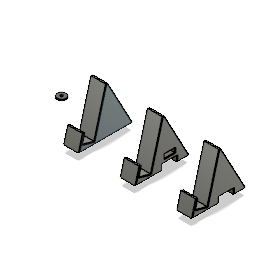
CD Jew Case Display Stand v5 (Autodesk Fusion 360 design; units mm, degrees)
Autodesk Fusion 360 part; units mm, degrees
sketch "Sketch1" plane through (0, 0, 0) normal (1, 0, 0) x (0, 0, -1)
  line L0 (0, 0) -> (-10.6, 0)
  line L1 (-10.6, 0) -> (-10.6, -2)
  line L2 (-10.6, -2) -> (0, -2)
  line L3 (0, -2) -> (0, 0)
  line L4 (-10.6, -2) -> (-12.6, -2)
  line L5 (-12.6, -2) -> (-12.6, 8)
  line L6 (-12.6, 8) -> (-10.6, 8)
  line L7 (-10.6, 8) -> (-10.6, -2)
  line L8 (0, -2) -> (2, -2)
  line L9 (2, -2) -> (2, 40)
  line L10 (2, 40) -> (0, 40)
  line L11 (0, 40) -> (0, -2)
  dimension "d1" = 10.6
  dimension "d2" = 2
  dimension "d3" = 2
  dimension "d4" = 10
  dimension "d5" = 2
  dimension "d6" = 42
  constraint horizontal L0
  constraint vertical L1
  constraint horizontal L2
  constraint vertical L3
  constraint coincident L0.start L3.end
  constraint horizontal L4
  constraint vertical L5
  constraint horizontal L6
  constraint vertical L7
  constraint horizontal L8
  constraint vertical L9
  constraint horizontal L10
  constraint vertical L11
  measures "d1" distance of L0.start L0.end
  measures "d2" distance of L0.start L2.end
  measures "d3" distance of L1.end L4.end
  measures "d4" distance of L1.end L6.end
  measures "d5" distance of L2.end L8.end
  measures "d6" distance of L2.end L10.end
extrude "Extrude1" add sketch "Sketch1" along normal blind 2 makes body 1
move_body "Move1" bodies 1 to x (1, 0, 0) y (0, 0.965926, -0.258819) z (0, 0.258819, 0.965926) at (0, 0.4495, -0.5858)
sketch "Sketch2" plane through (2, 0, 0) normal (1, 0, 0) x (0, 0, -1)
  line L0 (-12.1025, 1.7788) -> (2, -2)
  line L1 (2, -2) -> (12.8704, 38.5689)
  line L2 (12.8704, 38.5689) -> (10.9385, 39.0865)
  line L3 (10.9385, 39.0865) -> (0.5858, 0.4495)
  line L4 (0.5858, 0.4495) -> (-9.653, 3.193)
  line L5 (-9.653, 3.193) -> (-7.5825, 10.9204)
  line L6 (-7.5825, 10.9204) -> (-9.5143, 11.438)
  line L7 (-9.5143, 11.438) -> (-12.1025, 1.7788)
  line L8 (2, -2) -> (-13.115, -2)
  line L9 (-13.115, -2) -> (-12.1025, 1.7788)
  line L10 (2, -2) -> (32, -2)
  arc A0 (12.8704, 38.5689) -> (32, -2) centre (69.4566, 40.4566) ccw
  line L11 (12.8704, 38.5689) -> (32, -2)
  dimension "d9" = 30
  constraint coincident L0.end L1.start
  constraint horizontal L8
  constraint coincident L0.start L7.end
  constraint perpendicular L0 L9
  constraint horizontal L10
  constraint coincident L1.end L2.start
  measures "d9" distance of L0.end L10.end
extrude "Extrude2" add sketch "Sketch2" against normal blind 2 contours L0 L8 L9 | L1 L10 A0 | A0 L11 bodies 1
draft "Draft1" angle 3 neutral plane through (0, 38.5689, -12.8704) pull (0, 0.965926, -0.258819) 1 faces at (1.3333, 25.0459, -19.2469) on bodies 1
sketch "Sketch3" plane through (2, 0, 0) normal (1, 0, 0) x (0, 0, -1)
  line L0 (12.8704, 38.5689) -> (10.9385, 39.0865)
  line L1 (10.9385, 39.0865) -> (0.5858, 0.4495)
  line L2 (0.5858, 0.4495) -> (-9.653, 3.193)
  line L3 (-9.653, 3.193) -> (-7.5825, 10.9204)
  line L4 (-7.5825, 10.9204) -> (-9.5143, 11.438)
  line L5 (-9.5143, 11.438) -> (-13.115, -2)
  line L6 (-13.115, -2) -> (34.6647, -2)
  line L7 (34.6647, -2) -> (34.6647, 3)
  line L8 (34.6647, 3) -> (34.6647, 4)
  line L9 (34.6647, 4) -> (34.6647, 7.25)
  line L10 (34.6647, 7.25) -> (34.6647, 10.75)
  line L11 (34.6647, 10.75) -> (23.923, 10.75)
  line L12 (23.923, 10.75) -> (21.923, 10.75)
  line L13 (21.923, 10.75) -> (12.723, 10.75)
  line L14 (12.723, 10.75) -> (12.723, 7.25)
  line L15 (12.723, 7.25) -> (21.923, 7.25)
  line L16 (21.923, 7.25) -> (21.923, 10.75)
  line L17 (17.323, 7.25) -> (17.323, 4)
  line L18 (17.323, 4) -> (23.823, 4)
  line L19 (23.823, 4) -> (10.823, 4)
  line L20 (10.823, 4) -> (10.823, -2)
  line L21 (10.823, -2) -> (23.823, -2)
  line L22 (23.823, -2) -> (23.823, 4)
  line L23 (34.6647, -2) -> (12.8704, 38.5689)
  dimension "d12" = 5
  dimension "d13" = 3.25
  dimension "d14" = 3.5
  dimension "d15" = 2
  dimension "d16" = 9.2
  dimension "d17" = 3.5
  dimension "d18" = 3.25
  dimension "d19" = 6.5
  dimension "d20" = 13
  constraint coincident L6.end L7.start
  constraint perpendicular L6 L7
  constraint parallel L7 L8
  constraint parallel L8 L9
  constraint parallel L9 L10
  constraint perpendicular L10 L11
  constraint perpendicular L10 L12
  constraint horizontal L13
  constraint vertical L14
  constraint horizontal L15
  constraint vertical L16
  constraint midpoint L15 L17.start
  constraint perpendicular L15 L17
  constraint perpendicular L17 L18
  constraint horizontal L19
  constraint vertical L20
  constraint horizontal L21
  constraint vertical L22
  measures "d12" distance of L6.end L7.end
  measures "d13" distance of L8.end L9.end
  measures "d14" distance of L9.end L10.end
  measures "d15" distance of L11.end L12.end
  measures "d16" distance of L12.end L13.end
  measures "d17" distance of L12.end L15.end
  measures "d18" distance of L17.start L17.end
  measures "d19" distance of L17.end L18.end
  measures "d20" distance of L18.end L19.end
extrude "Extrude3" add 1 faces at (0, 12.3395, -16.0403) along direction (-1, 0, 0) blind 12 on bodies 1 bodies 1
copy_body "CopyPasteBodies1" bodies 1 makes body 2
move_body "Move2" bodies 2 to x (1, 0, 0) y (0, 1, 0) z (0, 0, 1) at (-50, 0, 0)
copy_body "CopyPasteBodies2" bodies 1 2 makes body 3 makes body 4
move_body "Move3" bodies 3 4 to x (1, 0, 0) y (0, 1, 0) z (0, 0, 1) at (-100, 0, 0)
extrude "Extrude4" cut sketch "Sketch3" against normal blind 64 contours L13 L14 L15 L16 | L6 L18 L19 L20 L21 L22 bodies 1 2
extrude "Extrude5" add sketch "Sketch3" against normal blind 2 contours L13 L14 L15 L16 bodies 1
extrude "Extrude6" add sketch "Sketch3" along normal blind -64 and the other way blind 62 contours L13 L14 L15 L16 bodies 2
sketch "Sketch4" plane through (0, 0, 0) normal (0, 1, 0) x (1, 0, 0)
  circle A0 centre (28.667, 5.442) radius 10.4527
  ellipse E0 centre (28.667, 5.442) end of major axis (31.6436, 5.442) minor radius 2.9766
  point P0 (39.1197, 5.442)
  point P1 (31.6436, 5.442)
extrude "Extrude7" add sketch "Sketch4" along normal blind 3 separate body makes body 5
scale "Scale1" factor 0.382665 about (39.1197, 0, -5.442) bodies 5
move_body "Move4" bodies 5 to x (1, 0, 0) y (0, 1, 0) z (0, 0, 1) at (-33.1198, -2, -23.8018)
move_body "Move5" bodies 5 to x (1, 0, 0) y (0, 1, 0) z (0, 0, 1) at (-7, -5, 0)
extrude "Extrude8" cut 1 faces at (-5, -5.852, -32.2827) along direction (0, 1, 0) blind 4.352 on bodies 5 bodies 1
extrude "Extrude9" cut 1 faces at (-5.3459, -2, -29.0223) along direction (0, 1, 0) blind 1 on bodies 1 bodies 1
move_body "Move6" bodies 5 to x (1, 0, 0) y (0, 1, 0) z (0, 0, 1) at (-43, 5, 0)
move_body "Move7" bodies 5 to x (1, 0, 0) y (0, 1, 0) z (0, 0, 1) at (-7, -5, 0)
extrude "Extrude10" cut 1 faces at (-55, -5.852, -32.2827) along direction (0, 1, 0) blind 4.352 on bodies 5 bodies 2
move_body "Move8" bodies 5 to x (1, 0, 0) y (0, 1, 0) z (0, 0, 1) at (-50, 5, -5.4209)
move_body "Move9" bodies 5 to x (1, 0, 0) y (0, 1, 0) z (0, 0, 1) at (0, -5, 6)
extrude "Extrude11" cut 1 faces at (-105, -5.852, -31.7035) along direction (0, 1, 0) blind 4.352 on bodies 5 bodies 3
move_body "Move10" bodies 5 to x (1, 0, 0) y (0, 1, 0) z (0, 0, 1) at (-50, 3.852, -6)
move_body "Move11" bodies 5 to x (1, 0, 0) y (0, 1, 0) z (0, 0, 1) at (0, -5, 6)
extrude "Extrude12" cut 1 faces at (-155, -7, -31.7035) along direction (0, 1, 0) blind 5.5 on bodies 5 bodies 4
extrude "Extrude13" cut 3 faces at (-155.3459, -2, -28.4431) (-105.3458, -2, -28.4429) (-55.3055, -2, -29.4529) along direction (0, 1, 0) blind 1 on bodies 2 3 4 bodies 2 3 4
delete_body "RemoveBody1" bodies 4
sketch "Sketch5" plane through (0, -2, 0) normal (0, -1, 0) x (1, 0, 0)
  line L0 (-62, -10.823) -> (-48, -10.823)
  line L1 (-48, -10.823) -> (-48, 13.115)
  line L2 (-48, 13.115) -> (-62, 13.115)
  line L3 (-62, 13.115) -> (-62, -10.823)
  line L4 (-62, 1.146) -> (-48, 1.146) construction
  line L5 (-48, 1.146) -> (-48, 13.115) construction
  line L6 (-48, 13.115) -> (-62, 13.115) construction
  line L7 (-62, 13.115) -> (-62, 1.146) construction
  text T0 "L" font "Arial" height 10 align centre middle in box 14 x 11.969 at (-62, 1.146) x (1, 0) y (0, 1) spacing 1 kerned
  constraint midpoint L1
  constraint coincident L2.end
sketch "Sketch6" plane through (0, -2, 0) normal (0, -1, 0) x (1, 0, 0)
  line L0 (-12, -10.823) -> (2, -10.823)
  line L1 (2, -10.823) -> (2, 13.115)
  line L2 (2, 13.115) -> (-12, 13.115)
  line L3 (-12, 13.115) -> (-12, -10.823)
  line L4 (-12, 1.146) -> (2, 1.146) construction
  line L5 (2, 1.146) -> (2, 13.115) construction
  line L6 (2, 13.115) -> (-12, 13.115) construction
  line L7 (-12, 13.115) -> (-12, 1.146) construction
  text T0 "R" font "Arial" height 10 align centre middle in box 14 x 11.969 at (-12, 1.146) x (1, 0) y (0, 1) spacing 1 kerned
  constraint midpoint L1
  constraint coincident L2.end
extrude "Extrude14" cut sketch "Sketch6" sketch "Sketch5" against normal blind 1 text T0 of sketch 2 text T0 bodies 1 2
sketch "Sketch7" plane through (0, 4, 0) normal (0, -1, 0) x (1, 0, 0)
  line L0 (-48, -23.823) -> (-48, -10.823)
  line L1 (-48, -10.823) -> (-62, -10.823)
  line L2 (-62, -10.823) -> (-62, -23.823)
  line L3 (-62, -23.823) -> (-48, -23.823)
  line L4 (-55, -10.823) -> (-55, -23.823)
  circle A0 centre (-55, -17.323) radius 2.4
  dimension "d50" = 4.8
  constraint midpoint L1 L4.start
  constraint midpoint L3 L4.end
  constraint midpoint L4 A0.centre
  measures "d50" diameter of A0
extrude "Extrude15" cut sketch "Sketch7" against normal blind 11 contours L4 A0 | L4 A0 bodies 2
sketch "Sketch8" plane through (0, 4, 0) normal (0, -1, 0) x (1, 0, 0)
  line L0 (-12, -10.823) -> (-12, -23.823)
  line L1 (-12, -23.823) -> (2, -23.823)
  line L2 (2, -23.823) -> (2, -10.823)
  line L3 (2, -10.823) -> (-12, -10.823)
  line L4 (-12, -17.323) -> (2, -17.323)
  circle A0 centre (-5, -17.323) radius 2.4
  dimension "d53" = 4.8
  constraint midpoint L0 L4.start
  constraint midpoint L2 L4.end
  constraint midpoint L4 A0.centre
  measures "d53" diameter of A0
extrude "Extrude16" cut sketch "Sketch8" against normal blind 11 contours L4 A0 | L4 A0 bodies 1
move_face "OffsetFaces1" offset -0.2 2 faces at (-52.6119, 5.0833, -17.562) (-2.603, 5.0833, -17.2034) on bodies 1 2
move_face "MoveFace1" by (0, -1, 0) 8 faces at (-10.5333, 4, -17.323) (-49.4667, 4, -17.323) (-49.5333, 10.75, -17.323) (-10.4667, 10.75, -17.323) (-10.5333, 7.25, -17.323) (-49.4667, 7.25, -17.323) (-5.0792, 15, -16.7846) (-55.4105, 15, -18.0855) on bodies 1 2
chamfer "Chamfer1" distance 0.5 angle 45 5 faces at (-48, 16.4287, -8.0824) (-62, 14.8563, -15.8388) (-98, 12.3395, -16.0403) (2, 14.8563, -15.8388) (-12, 16.4287, -8.0824) on bodies 1 2 3
chamfer "Chamfer2" distance 0.5 angle 45 1 faces at (-112, 12.3395, -16.0403) on bodies 3
sketch "Sketch9" plane through (-98, 0, 0) normal (1, 0, 0) x (0, 0, -1)
  line L0 (-12.4634, -1.5) -> (33.8285, -1.5)
  line L1 (33.8285, -1.5) -> (12.5322, 38.1419)
  line L2 (12.5322, 38.1419) -> (11.2921, 38.4742)
  line L3 (11.2921, 38.4742) -> (0.9393, -0.1629)
  line L4 (0.9393, -0.1629) -> (-10.2654, 2.8394)
  line L5 (-10.2654, 2.8394) -> (-8.1948, 10.5668)
  line L6 (-8.1948, 10.5668) -> (-9.1608, 10.8256)
  line L7 (-9.1608, 10.8256) -> (-12.4634, -1.5)
equation "d19 = ( 13 / 2 ) * 1 mm"
equation "d21 = -2 mm + 14 mm"
equation "d29 = 64.00 mm - 2 mm"
equation "d35 = 8 / 20.906"
equation "d36 = 3.852 mm + 0.5 mm"
equation "d40 = 3.852 mm + 0.5 mm"
equation "d42 = 3.852 mm + 0.5 mm"
equation "d44 = 5.00 mm + 0.5 mm"
named bodies: "CD Kit Right", "CD Kit Left", "CD Leg", "DVD Icon"
